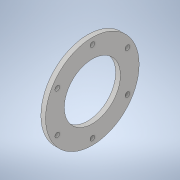
# Autodesk Inventor part: BearingAdapter
Saved by Autodesk Inventor 2021 (Build 250183000, 183)
## iProperties
Created: 2020-09-20
Part Number: BearingAdapter
Material: Generic
Document SubType Name: Modeling
Designer: PhotonUser
Density: 1 g/cm^3
Appearance: Default
Author: PhotonUser
Autodesk Inventor part; units mm, degrees
ref_plane "YZ Plane" through (0, 0, 0) normal (1, 0, 0) x (0, 1, 0)
ref_plane "XZ Plane" through (0, 0, 0) normal (0, 1, 0) x (-1, 0, 0)
ref_plane "XY Plane" through (0, 0, 0) normal (0, 0, 1) x (1, 0, 0)
sketch "Sketch1" plane through (0, 0, 0) normal (1, 0, 0) x (0, 1, 0)
  circle A0 centre (0, 0) radius 63.5
  circle A1 centre (55.0037, 0) radius 3.175
  line L0 (0, 0) -> (83.9398, 0)
  circle A2 centre (27.5019, -47.6346) radius 3.175
  circle A3 centre (-27.5018, -47.6346) radius 3.175
  circle A4 centre (-55.0037, 0) radius 3.175
  circle A5 centre (-27.5019, 47.6346) radius 3.175
  circle A6 centre (27.5018, 47.6346) radius 3.175
  dimension "d0" = 127
  dimension "d1" = 6.35
  dimension "d2" = 55.0037
  dimension "d5" = 360
  constraints: 7 centre point, 3 coincident, 2 end point, 1 horizontal, 1 point on line, 17 other
  measures "d0" diameter of A0
  measures "d1" diameter of A1
  measures "d2" distance of A1.centre point (0, 0)
extrude "Extrusion1" add sketch "Sketch1" along normal blind 6.35
sketch "Sketch2" plane through (6.35, 0, 0) normal (1, 0, 0) x (0, 0, -1)
  circle A0 centre (0, 0) radius 38.1
  dimension "d9" = 76.2
  constraints: 1 centre point, 1 coincident
  measures "d9" diameter of A0
extrude "Extrusion2" cut sketch "Sketch2" against normal blind 6.35
body "Solid1"
